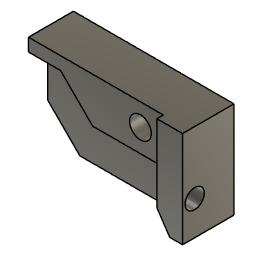
task 1 v1 (Autodesk Fusion 360 design; units mm, degrees)
Autodesk Fusion 360 part; units mm, degrees
sketch "Sketch1" plane through (0, 0, 0) normal (0, 1, 0) x (1, 0, 0)
  line L0 (0, 0) -> (0, 50)
  line L1 (0, 0) -> (0, 50)
  line L2 (0, 50) -> (25, 75)
  line L3 (25, 75) -> (100, 75)
  line L4 (100, 0) -> (0, 0)
  line L5 (100, 0) -> (125, 0)
  line L6 (125, 0) -> (125, 75)
  line L7 (125, 75) -> (100, 75)
  constraint coincident L0.start L1.start
  constraint vertical L0
  constraint perpendicular L1 L3
  constraint perpendicular L0 L4
  constraint parallel L4 L5
  constraint perpendicular L5 L6
  constraint perpendicular L6 L7
extrude "Extrude1" add sketch "Sketch1" along normal blind 20
sketch "Sketch2" plane through (0, 0, 0) normal (0, -1, 0) x (1, 0, 0)
  line L0 (125, 0) -> (0, 0)
  line L1 (0, 0) -> (0, -50)
  line L2 (0, -50) -> (25, -75)
  line L3 (25, -75) -> (125, -75)
  line L4 (125, -75) -> (125, 0)
  line L5 (125, 0) -> (105, 0)
  line L6 (105, -60) -> (115, -75)
  line L7 (105, -60) -> (105, 0)
  line L8 (125, 0) -> (125, -75)
  constraint coincident L0.start L4.end
  constraint coincident L0 L5.end
  constraint coincident L3 L6.end
  constraint perpendicular L5 L7
  constraint coincident L4 L3.end
extrude "Extrude2" add sketch "Sketch2" along normal blind 20 contours L0 L3 L4 L5 L6 L7 L8
sketch "Sketch3" plane through (0, 0, 0) normal (0, -1, 0) x (1, 0, 0)
  line L0 (115, -75) -> (105, -60)
  line L1 (105, -60) -> (105, 0)
  line L2 (105, 0) -> (0, 0)
  line L3 (0, 0) -> (0, -50)
  line L4 (0, -50) -> (25, -75)
  line L5 (25, -75) -> (115, -75)
  line L6 (0, -10) -> (25, -10)
  line L7 (25, -10) -> (50, -35)
  line L8 (50, -35) -> (105, -35)
  line L9 (105, 0) -> (0, 0)
  constraint coincident L3 L6.start
  constraint perpendicular L3 L6
  constraint coincident L1 L8.end
  constraint perpendicular L1 L8
  constraint coincident L1.end L2.start
  constraint coincident L2.end L3.start
extrude "Extrude3" add sketch "Sketch3" along normal blind 15 contours L1 L2 L3 L6 L7 L8 L9
sketch "Sketch4" plane through (0, -15, 0) normal (0, -1, 0) x (1, 0, 0)
  line L0 (105, 0) -> (0, 0)
  line L1 (0, 0) -> (0, -10)
  line L2 (0, -10) -> (25, -10)
  line L3 (25, -10) -> (50, -35)
  line L4 (50, -35) -> (105, -35)
  line L5 (105, -35) -> (105, 0)
  circle A0 centre (87.1903, -17.2532) radius 8.5
  dimension "d7" = 17
  measures "d7" diameter of A0
hole "Hole1" at (87.1903, -15, -17.2532) direction (0, 1, 0) diameter 17 depth 35 tip angle 180
sketch "Sketch5" plane through (0, -20, 0) normal (0, -1, 0) x (1, 0, 0)
  line L0 (105, -60) -> (115, -75)
  line L1 (115, -75) -> (125, -75)
  line L2 (125, -75) -> (125, 0)
  line L3 (125, 0) -> (105, 0)
  line L4 (105, 0) -> (105, -60)
  circle A0 through (105, -41.1018, -9.4428) (105, -52.3518, -2.9476) (105, -52.3518, -15.938)
  dimension "d13" = 15
extrude "Extrude4" cut sketch "Sketch5" against normal blind -20 and the other way blind 0 contours A0 in plane through (105, -20, 0) normal (1, 0, 0)
